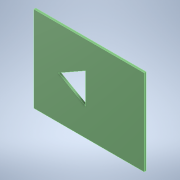
# Autodesk Inventor part: PCB-main
Saved by Autodesk Inventor 2022 (Build 260153000, 153)
## iProperties
Created: 2024-06-04
Part Number: PCB-main
Material: 一般
Document SubType Name: Modeling
Designer: yamashita1
Density: 1 g/cm^3
Appearance: 滑らか - 濃い深緑
Author: yamashita1
Autodesk Inventor part; units mm, degrees
ref_plane "YZ Plane" through (0, 0, 0) normal (1, 0, 0) x (0, 1, 0)
ref_plane "XZ Plane" through (0, 0, 0) normal (0, 1, 0) x (-1, 0, 0)
ref_plane "XY Plane" through (0, 0, 0) normal (0, 0, 1) x (1, 0, 0)
sketch "スケッチ1" plane through (0, 0, 0) normal (0, 0, 1) x (1, 0, 0)
  line L0 (-45, 35) -> (45, 35)
  line L1 (45, 35) -> (45, -35)
  line L2 (45, -35) -> (-45, -35)
  line L3 (-45, -35) -> (-45, 35)
  point P0 (0, 0)
  point P1 (-45, 0)
  point P2 (0, 35)
  dimension "d0" = 90
  dimension "d1" = 70
  constraints: 8 end point, 2 midpoint, 2 parallel, 1 horizontal, 1 horizontal alignment, 1 perpendicular, 1 vertical alignment
  measures "d0" distance of L1.end L2.end
  measures "d1" distance of L0.end L1.end
extrude "押し出し1" add sketch "スケッチ1" along normal blind 1.6
sketch "スケッチ2" plane through (0, 0, 1.6) normal (0, 0, 1) x (1, 0, 0)
  line L0 (-25, 0) -> (-3, -12.5)
  line L1 (-3, -12.5) -> (-3, 12.5)
  line L2 (-3, 12.5) -> (-25, 0)
  line L3 (-45, 35) -> (-45, -35) projected
  point P0 (0, 0)
  point P1 (-3, 0)
  dimension "d4" = 25
  dimension "d5" = 22
  dimension "d6" = 20
  constraints: 6 end point, 2 horizontal alignment, 1 midpoint, 1 vertical
  measures "d4" distance of L0.end L1.end
  measures "d5" distance from line of L0.start L1
  measures "d6" distance from line of L3 L0.start
extrude "押し出し2" cut sketch "スケッチ2" against normal through all
